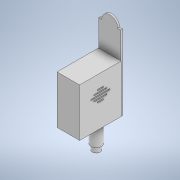
# Autodesk Inventor part: endeffector_30mm
Saved by Autodesk Inventor 2022 (Build 260153000, 153)
## iProperties
Created: 2023-01-13
Part Number: endeffector_30mm
Material: 一般
Document SubType Name: Modeling
Designer: TingWeiOu
Density: 1 g/cm^3
Appearance: 預設
Author: TingWeiOu
Autodesk Inventor part; units mm, degrees
ref_plane "YZ Plane" through (0, 0, 0) normal (1, 0, 0) x (0, 1, 0)
sketch "草圖1" plane through (0, 0, 0) normal (1, 0, 0) x (0, 1, 0)
  line L0 (-90.5, -78) -> (90.5, -78)
  line L1 (90.5, -78) -> (90.5, 78)
  line L2 (90.5, 78) -> (-90.5, 78)
  line L3 (-90.5, 78) -> (-90.5, -78)
  line L4 (-90.5, -78) -> (90.5, 78) construction
  line L5 (90.5, -78) -> (-90.5, 78) construction
  point P0 (0, 0)
  dimension "d0" = 156
  dimension "d1" = 181
  constraints: 12 end point, 2 midpoint, 2 parallel, 1 horizontal, 1 perpendicular
  measures "d0" distance of L0.end L1.end
  measures "d1" distance of L0.start L0.end
extrude "擠出1" add sketch "草圖1" along normal mid plane 85
ref_plane "工作平面1" through (-42.5, -196.5, 78) normal (0, 1, 0) x (1, 0, 0)
sketch "草圖2" plane through (-42.5, -90.5, -78) normal (0, -1, 0) x (1, 0, 0)
  circle A0 centre (42.5, 51) radius 20
  line L0 (0, 156) -> (85, 156) projected
  point P0 (42.5, 78)
  dimension "d5" = 105
  dimension "d8" = 40
  constraints: 1 centre point
  measures "d5" distance from line of L0 A0.centre
  measures "d8" diameter of A0
extrude "擠出2" add sketch "草圖2" along normal blind 85
sketch "草圖3" plane through (-42.5, -90.5, -78) normal (0, -1, 0) x (1, 0, 0)
  circle A0 centre (42.5, 51) radius 20 projected
  circle A1 centre (42.5, 51) radius 29.5638
  point P0 (42.5, 78)
  constraints: 1 centre point, 1 coincident
extrude "擠出3" add sketch "草圖3" along normal blind 2
sketch "草圖4" plane through (0, -175.5, -27) normal (0, -1, 0) x (1, 0, 0)
  circle A0 centre (0, 0) radius 20 projected
  circle A1 centre (0, 0) radius 15
  point P0 (0, 27)
  dimension "d11" = 30
  constraints: 1 centre point, 1 coincident
  measures "d11" diameter of A1
extrude "擠出4" add sketch "草圖4" along normal up to surface (21 mm away) contours A1
sketch "草圖5" plane through (0, 0, 0) normal (1, 0, 0) x (0, 1, 0)
  point P0 (0, 0)
fillet "圓角1" radius 2 1 edges at (-15, -196.5, -27)
fillet "圓角2" radius 2 3 edges at (-15, -175.5, -27) (-20, -175.5, -27) (-20, -92.5, -27)
sketch "草圖6" plane through (42.5, 0, 0) normal (1, 0, 0) x (0, 0, -1)
  line L0 (-34.1429, 20) -> (34.1429, 20) construction
  line L1 (-34.1429, 18) -> (34.1429, 18)
  line L2 (34.1429, 22) -> (-34.1429, 22)
  arc A0 (-34.1429, 22) -> (-34.1429, 18) centre (-34.1429, 20) ccw
  arc A1 (34.1429, 18) -> (34.1429, 22) centre (34.1429, 20) ccw
  line L3 (0, 0) -> (0, 59.057)
  line L4 (-22.9286, 30) -> (22.9286, 30) construction
  line L5 (-22.9286, 28) -> (22.9286, 28)
  line L6 (22.9286, 32) -> (-22.9286, 32)
  arc A2 (-22.9286, 32) -> (-22.9286, 28) centre (-22.9286, 30) ccw
  arc A3 (22.9286, 28) -> (22.9286, 32) centre (22.9286, 30) ccw
  line L7 (-10, 40) -> (10, 40) construction
  line L8 (-10, 38) -> (10, 38)
  line L9 (10, 42) -> (-10, 42)
  arc A4 (-10, 42) -> (-10, 38) centre (-10, 40) ccw
  arc A5 (10, 38) -> (10, 42) centre (10, 40) ccw
  point P0 (0, 20)
  point P1 (0, 30)
  point P2 (0, 40)
  dimension "d16" = 2
  dimension "d17" = 2
  dimension "d18" = 2
  dimension "d19" = 10
  dimension "d20" = 10
  dimension "d23" = 20
  dimension "d24" = 20
  constraints: 26 end point, 12 point on circle, 12 tangent, 6 centre point, 4 parallel, 3 midpoint, 3 symmetric about line, 2 horizontal, 1 vertical
  measures "d16" radius of A0
  measures "d17" radius of A2
  measures "d18" radius of A4
  measures "d19" distance of point (0, 20) point (0, 30)
  measures "d20" distance of point (0, 40) point (0, 30)
  measures "d23" distance of L7.end L7.start
  measures "d24" distance of L3.start point (0, 20)
extrude "擠出5" cut sketch "草圖6" against normal blind 10
ref_plane "工作平面2" through (0, 20, 0) normal (0, 1, 0) x (-1, 0, 0)
mirror "鏡射1" about plane through (0, 20, 0) normal (0, 1, 0) of "擠出5"
sketch "草圖7" plane through (42.5, 90.5, -78) normal (0, 0, -1) x (-1, 0, 0)
  line L0 (85, -181) -> (0, -181) projected
  line L1 (1, -181) -> (84, -181)
  line L2 (84, -181) -> (84, 100)
  line L3 (84, 100) -> (1, 100)
  line L4 (1, 100) -> (1, -181)
  line L5 (0, -181) -> (0, 0) projected
  line L6 (85, 0) -> (85, -181) projected
  line L7 (0, 0) -> (85, 0) projected
  point P0 (42.5, -90.5)
  dimension "d26" = 1
  dimension "d27" = 1
  dimension "d28" = 100
  constraints: 8 end point, 2 parallel, 1 horizontal, 1 perpendicular, 1 point on line
  measures "d26" distance between parallel lines of L4 L5
  measures "d27" distance between parallel lines of L6 L2
  measures "d28" distance between parallel lines of L7 L3
extrude "擠出6" add sketch "草圖7" along normal blind 7 contours L0 L4 L7 L2 | L7 L4 L3 L2
sketch "草圖8" plane through (42.5, 90.5, -85) normal (0, 0, -1) x (-1, 0, 0)
  line L0 (84, 100) -> (1, 100) projected
  circle A0 centre (42.5, 100) radius 30
  point P0 (42.5, -90.5)
  point P1 (12.5, 100)
  point P2 (72.5, 100)
  dimension "d31" = 60
  constraints: 1 centre point, 1 midpoint
  measures "d31" diameter of A0
extrude "擠出7" add sketch "草圖8" against normal blind 7 contours L0 A0 picked at (46.046, 109.3502)
equation "\"d21\" = d19"
